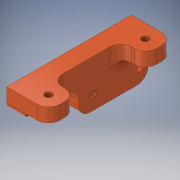
# Autodesk Inventor part: EquerrePCBDroite
Saved by Autodesk Inventor 2019 (Build 230136000, 136)
## iProperties
Created: 2019-07-30
Part Number: EquerrePCBDroite
Material: Plastique ABS
Document SubType Name: Modeling
Designer: Sébastien DI MERCURIO
Mass: 12.1635 g
Surface Area: 33.9 cm^2
Volume: 11.475 cm^3
Density: 1.06 g/cm^3
Appearance: Lisse - Orange clair
Author: Sébastien DI MERCURIO
Autodesk Inventor part; units mm, degrees
ref_plane "YZ Plane" through (0, 0, 0) normal (1, 0, 0) x (0, 1, 0)
ref_plane "XZ Plane" through (0, 0, 0) normal (0, 1, 0) x (-1, 0, 0)
ref_plane "XY Plane" through (0, 0, 0) normal (0, 0, 1) x (1, 0, 0)
sketch "Esquisse1" plane through (0, 0, 0) normal (0, 0, 1) x (1, 0, 0)
  line L0 (0, 0) -> (15, 0)
  line L1 (15, 0) -> (15, 17)
  line L2 (15, 17) -> (0, 17)
  line L3 (0, 17) -> (0, 0)
  dimension "d0" = 15
  dimension "d1" = 17
  constraints: 8 end point, 2 parallel, 1 horizontal, 1 perpendicular
  measures "d0" distance of L1.end L2.end
  measures "d1" distance of L0.end L1.end
extrude "Extrusion1" add sketch "Esquisse1" along normal blind 45
sketch "Esquisse2" plane through (0, 0, 45) normal (0, 0, 1) x (1, 0, 0)
  line L0 (0, 0) -> (15, 0) projected
  line L1 (15, 0) -> (6, 0)
  line L2 (6, 0) -> (6, 12)
  line L3 (6, 12) -> (15, 12)
  line L4 (15, 12) -> (15, 0)
  line L5 (15, 17) -> (0, 17) projected
  line L6 (0, 17) -> (0, 0) projected
  dimension "d4" = 5
  dimension "d5" = 6
  constraints: 8 end point, 2 parallel, 1 horizontal, 1 perpendicular
  measures "d4" distance between parallel lines of L3 L5
  measures "d5" distance between parallel lines of L6 L2
extrude "Extrusion2" cut sketch "Esquisse2" against normal through all
sketch "Esquisse3" plane through (0, 17, 0) normal (0, 1, 0) x (1, 0, 0)
  line L0 (15, 0) -> (15, -45) projected
  line L1 (15, -35) -> (6, -35)
  line L2 (6, -35) -> (6, -10)
  line L3 (6, -10) -> (15, -10)
  line L4 (15, -10) -> (15, -35)
  line L5 (15, -45) -> (0, -45) projected
  line L6 (15, 0) -> (0, 0) projected
  line L7 (0, 0) -> (0, -45) projected
  dimension "d8" = 25
  dimension "d9" = 45
  dimension "d10" = 10
  dimension "d11" = 6
  constraints: 8 end point, 2 parallel, 1 horizontal, 1 perpendicular, 1 point on line
  measures "d8" distance of L1.end L2.end
  measures "d9" distance between parallel lines of L5 L6
  measures "d10" distance between parallel lines of L6 L3
  measures "d11" distance between parallel lines of L7 L2
extrude "Extrusion3" cut sketch "Esquisse3" against normal through all contours L0 L1 L2 L3
sketch "Esquisse5" plane through (0, 0, 45) normal (-1, 0, 0) x (0, 0, 1)
  circle A0 centre (-42, 5) radius 1.25
  circle A1 centre (-25, 5) radius 1.25
  line L0 (0, 17) -> (0, 0) projected
  line L1 (-45, 0) -> (0, 0) projected
  line L2 (-45, 17) -> (-45, 0) projected
  point P0 (-25, 0)
  dimension "d18" = 2.5
  dimension "d19" = 17
  dimension "d21" = 5
  dimension "d33" = 3
  constraints: 2 centre point, 1 equal radius, 1 horizontal alignment
  measures "d18" diameter of A0
  measures "d19" distance of A1.centre A0.centre
  measures "d21" distance from line of L1 A0.centre
  measures "d33" distance from line of L2 A0.centre
extrude "Extrusion5" cut sketch "Esquisse5" against normal through all
sketch "Esquisse6" plane through (0, 17, 0) normal (0, 1, 0) x (1, 0, 0)
  circle A0 centre (10, -5) radius 1.25
  circle A1 centre (10, -40) radius 1.25
  line L0 (15, 0) -> (0, 0) projected
  line L1 (15, -45) -> (0, -45) projected
  line L2 (15, 0) -> (15, -10) projected
  dimension "d24" = 2.5
  dimension "d25" = 5
  dimension "d26" = 5
  dimension "d27" = 5
  constraints: 2 centre point, 1 equal radius, 1 vertical alignment
  measures "d24" diameter of A0
  measures "d25" distance from line of A0.centre L0
  measures "d26" distance from line of L1 A1.centre
  measures "d27" distance from line of L2 A0.centre
extrude "Extrusion6" cut sketch "Esquisse6" against normal through all
sketch "Esquisse7" plane through (0, 0, 0) normal (-1, 0, 0) x (0, 0, 1)
  line L0 (45, 17) -> (45, 0) projected
  line L1 (45, 0) -> (25, 0)
  line L2 (25, 0) -> (25, 10)
  line L3 (25, 10) -> (45, 10)
  line L4 (45, 10) -> (45, 0)
  point P0 (0, 0)
  dimension "d34" = 20
  dimension "d35" = 10
  constraints: 8 end point, 2 parallel, 1 horizontal, 1 perpendicular
  measures "d34" distance of L2.end L3.end
  measures "d35" distance of L0.end L3.end
extrude "Extrusion7" cut sketch "Esquisse7" against normal through all
fillet "Congé1" radius 4 6 edges at (15, 14.5, 10) (15, 14.5, 0) (15, 14.5, 35) (15, 14.5, 45) (6, 14.5, 35) (6, 14.5, 10)
fillet "Congé4" radius 4 3 edges at (3, 0, 25) (3, 10, 25) (3, 0, 0)
fillet "Congé5" radius 2 1 edges at (3, 10, 45)
fillet "Congé6" radius 2 4 edges at (6, 12, 40) (6, 12, 33) (6, 12, 12) (6, 12, 5)
equation "\"d10\" = -0.5 * d8 + 0.5 * d9"
